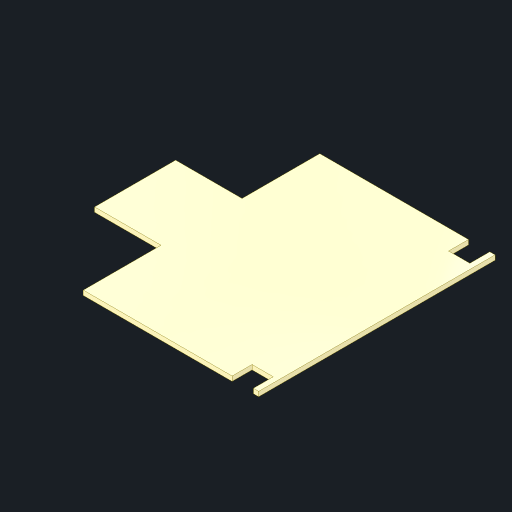
# Autodesk Inventor part: base
Saved by Autodesk Inventor 2023 (Build 270158000, 158)
## iProperties
Created: 2024-04-29
Part Number: base
Material: Nylon 6/6
Document SubType Name: Modeling
Designer: szymo
Density: 1.13 g/cm^3
Appearance: Nylon 6
Mass: 104.475 g
Surface Area: 555.62 cm^2
Volume: 92.456 cm^3
Author: szymo
Autodesk Inventor part; units mm, degrees
ref_plane "YZ Plane" through (0, 0, 0) normal (1, 0, 0) x (0, 1, 0)
ref_plane "XZ Plane" through (0, 0, 0) normal (0, 1, 0) x (-1, 0, 0)
ref_plane "XY Plane" through (0, 0, 0) normal (0, 0, 1) x (1, 0, 0)
sketch "Sketch1" plane through (0, 0, 0) normal (0, 1, 0) x (-1, 0, 0)
  line L0 (99, 89) -> (-99, 89)
  line L1 (-99, 89) -> (-99, -89)
  line L2 (-99, -89) -> (99, -89)
  line L3 (99, -89) -> (99, 89)
  line L4 (99, 89) -> (-99, -89) construction
  line L5 (-99, 89) -> (99, -89) construction
  line L6 (-99, 89) -> (-85, 89)
  line L7 (-85, 89) -> (-85, -89)
  line L8 (-85, -89) -> (-99, -89)
  line L9 (-99, -89) -> (-99, 89)
  line L10 (99, 89) -> (97, 89)
  line L11 (97, 89) -> (97, -89)
  line L12 (97, -89) -> (99, -89)
  line L13 (99, -89) -> (99, 89)
  line L14 (97, 33) -> (97, 35)
  line L15 (97, -33) -> (97, -35)
  line L16 (97, 32.8) -> (97, 35)
  line L17 (97, -32.8) -> (97, -35)
  line L18 (97, 89) -> (47, 89)
  line L19 (47, 89) -> (47, 30.5)
  line L20 (47, 30.5) -> (97, 30.5)
  line L21 (97, 30.5) -> (97, 89)
  line L22 (97, -89) -> (47, -89)
  line L23 (47, -89) -> (47, -30.5)
  line L24 (47, -30.5) -> (97, -30.5)
  line L25 (97, -30.5) -> (97, -89)
  line L26 (-81, 74) -> (-81, 89) projected
  line L27 (-81, 31) -> (-81, 55) projected
  line L28 (-81, -12) -> (-81, 12) projected
  line L29 (-81, -55) -> (-81, -31) projected
  line L30 (-81, -89) -> (-81, -74) projected
  arc A0 (-81, 74) -> (-79, 72) centre (-79, 74) ccw projected
  line L31 (-70, 72) -> (-79, 72) projected
  line L32 (-70, 57) -> (-70, 72) projected
  line L33 (-79, 57) -> (-70, 57) projected
  arc A1 (-79, 57) -> (-81, 55) centre (-79, 55) ccw projected
  arc A2 (-81, 31) -> (-79, 29) centre (-79, 31) ccw projected
  line L34 (-70, 29) -> (-79, 29) projected
  line L35 (-70, 14) -> (-70, 29) projected
  line L36 (-79, 14) -> (-70, 14) projected
  arc A3 (-79, 14) -> (-81, 12) centre (-79, 12) ccw projected
  arc A4 (-81, -12) -> (-79, -14) centre (-79, -12) ccw projected
  line L37 (-70, -14) -> (-79, -14) projected
  line L38 (-70, -29) -> (-70, -14) projected
  line L39 (-79, -29) -> (-70, -29) projected
  arc A5 (-79, -29) -> (-81, -31) centre (-79, -31) ccw projected
  arc A6 (-81, -55) -> (-79, -57) centre (-79, -55) ccw projected
  line L40 (-70, -57) -> (-79, -57) projected
  line L41 (-70, -72) -> (-70, -57) projected
  line L42 (-79, -72) -> (-70, -72) projected
  arc A7 (-79, -72) -> (-81, -74) centre (-79, -74) ccw projected
  circle A8 centre (-77, -64.5) radius 1.2295 projected
  circle A9 centre (-77, -21.5) radius 1.2295 projected
  circle A10 centre (-77, 21.5) radius 1.2295 projected
  circle A11 centre (-77, 64.5) radius 1.2295 projected
  line L43 (-65, 89) -> (-79, 89)
  line L44 (-79, 89) -> (-79, 75)
  line L45 (-79, 75) -> (-65, 75)
  line L46 (-65, 75) -> (-65, 89)
  line L47 (-65, 89) -> (-81, 89)
  line L48 (-81, 89) -> (-81, 74)
  line L49 (-81, 74) -> (-65, 74)
  line L50 (-65, 74) -> (-65, 89)
  line L51 (-99, 0) -> (97, 0)
  line L52 (0, 0) -> (-99, 0) construction
  line L53 (-65, -89) -> (-79, -89)
  line L54 (-79, -89) -> (-79, -75)
  line L55 (-79, -75) -> (-65, -75)
  line L56 (-65, -75) -> (-65, -89)
  line L57 (-65, -89) -> (-81, -89)
  line L58 (-81, -89) -> (-81, -74)
  line L59 (-81, -74) -> (-65, -74)
  line L60 (-65, -74) -> (-65, -89)
  line L61 (77.5, 29.5) -> (66.5, 29.5) projected
  line L62 (66.5, -29.5) -> (77.5, -29.5) projected
  point P0 (47, 89)
  point P1 (47, -89)
  point P2 (97, -30.5)
  point P3 (97, 30.5)
  point P4 (-81, -89)
  point P5 (-79, -74)
  dimension "d0" = 198
  dimension "d1" = 178
  dimension "d2" = 14
  dimension "d3" = 2
  dimension "d16" = 50
  dimension "d17" = 58.5
  dimension "d18" = 50
  dimension "d19" = 58.5
  dimension "d22" = 14
  dimension "d23" = 14
  dimension "d24" = 2
  dimension "d25" = 1
  dimension "d26" = 2
  dimension "d87" = 1
  dimension "d88" = 1
  constraints: 88 end point, 14 parallel, 10 symmetric about line, 8 perpendicular, 8 point on line, 7 horizontal, 4 midpoint, 2 collinear
  measures "d0" distance of L2.end L1.end
  measures "d1" distance of L1.end L0.end
  measures "d2" distance of L7.end L8.end
  measures "d3" distance of L12.end L11.end
  measures "d16" distance of L20.end L19.end
  measures "d17" distance of L19.end L18.end
  measures "d18" distance of L23.end L24.end
  measures "d19" distance of L22.end L23.end
  measures "d22" distance of L45.end L44.end
  measures "d23" distance of L44.end L43.end
  measures "d24" distance between parallel lines of L26 L44
  measures "d25" distance between parallel lines of L45 L49
  measures "d26" distance between parallel lines of L31 L49
  measures "d87" distance between parallel lines of L20 L61
  measures "d88" distance between parallel lines of L24 L62
extrude "Extrusion1" add sketch "Sketch1" along normal blind 3.5 contours L19 L20 L11 L51 L28 A3 L36 L35 L34 A2 L27 A1 L33 L32 L31 A0 L49 L50 L46 L0 | L2 L56 L60 L59 A7 L42 L41 L40 A6 L29 A5 L39 L38 L37 A4 L28 L51 L11 L24 L23 | L26 A0 L31 L32 L33 A1 L27 A2 L34 L35 L36 A3 L28 L51 L7 L0 | L28 A4 L37 L38 L39 A5 L29 A6 L40 L41 L42 A7 L30 L2 L7 L51 | A8 | A9 | A10 | A11
body "Solid1"
